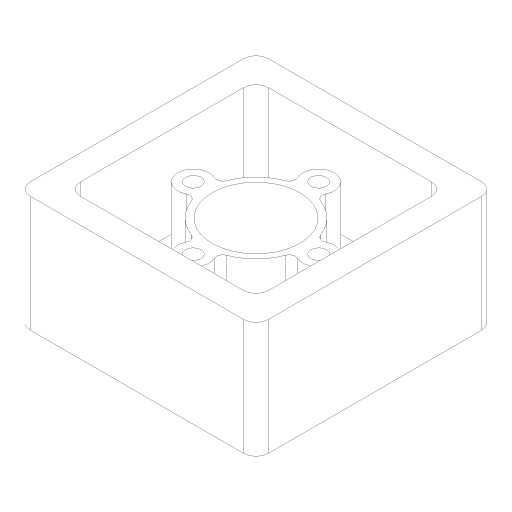
# Autodesk Inventor part: Ecoflex_mould
Saved by Autodesk Inventor 2023 (Build 270158000, 158)
## iProperties
Created: 2026-03-05
Part Number: Ecoflex_mould
Material: Generic
Document SubType Name: Modeling
Designer: ferrerx
Density: 1 g/cm^3
Appearance: Default
Author: ferrerx
Autodesk Inventor part; units mm, degrees
ref_plane "YZ Plane" through (0, 0, 0) normal (1, 0, 0) x (0, 1, 0)
ref_plane "XZ Plane" through (0, 0, 0) normal (0, 1, 0) x (-1, 0, 0)
ref_plane "XY Plane" through (0, 0, 0) normal (0, 0, 1) x (1, 0, 0)
sketch "Sketch1" plane through (0, 0, 0) normal (0, 1, 0) x (-1, 0, 0)
  circle A0 centre (0, 0) radius 7
  circle A1 centre (0, 0) radius 8
  dimension "d0" = 14
  dimension "d1" = 1
  constraints: 2 centre point, 2 coincident
  measures "d0" diameter of A0
  measures "d1" radial gap between concentric circles of A0 A1
extrude "Extrusion1" add sketch "Sketch1" along normal blind 10.5
sketch "Sketch2" plane through (0, 0, 0) normal (0, -1, 0) x (1, 0, 0)
  circle A0 centre (0, 0) radius 8
  constraints: 1 centre point, 1 coincident
extrude "Extrusion2" [suppressed]
sketch "Sketch4" plane through (0, 10.5, 0) normal (0, 1, 0) x (1, 0, 0)
  circle A0 centre (-10, 0) radius 1.25
  circle A1 centre (-10, 0) radius 2.5
  point P0 (0, 0)
  dimension "d6" = 5
  dimension "d7" = 2.5
  dimension "d8" = 10
  constraints: 2 centre point, 1 coincident
  measures "d6" diameter of A1
  measures "d7" diameter of A0
  measures "d8" distance of point (0, 0) A1.centre
extrude "Extrusion3" add sketch "Sketch4" against normal up to surface (10.5 mm away)
pattern_circular "Circular Pattern1" count 4 over 360 about axis through (0, 0, 0) along (0, 1, 0) of "Extrusion3"
fillet "Fillet1" radius 1 8 edges at (7.8875, 5.25, -1.3369) (7.8875, 5.25, 1.3369) (1.3369, 5.25, 7.8875) (-1.3369, 5.25, 7.8875) (-7.8875, 5.25, 1.3369) (-7.8875, 5.25, -1.3369) (-1.3369, 5.25, -7.8875) (1.3369, 5.25, -7.8875)
sketch "Sketch5" plane through (0, 0, 0) normal (0, -1, 0) x (1, 0, 0)
  line L0 (-15, -15) -> (15, -15)
  line L1 (15, -15) -> (15, 15)
  line L2 (15, 15) -> (-15, 15)
  line L3 (-15, 15) -> (-15, -15)
  line L4 (-15, -15) -> (15, 15) construction
  line L5 (15, -15) -> (-15, 15) construction
  point P0 (0, 0)
  dimension "d23" = 30
  dimension "d24" = 30
  constraints: 12 end point, 2 midpoint, 2 parallel, 1 horizontal, 1 perpendicular
  measures "d23" distance of L0.end L1.end
  measures "d24" distance of L0.start L0.end
extrude "Extrusion4" add sketch "Sketch5" along normal blind 4
sketch "Sketch6" plane through (0, -4, 0) normal (0, 1, 0) x (1, 0, 0)
  line L0 (15, 15) -> (15, -15) projected
  line L1 (-15, -15) -> (15, -15)
  line L2 (15, -15) -> (15, 15)
  line L3 (15, 15) -> (-15, 15)
  line L4 (-15, 15) -> (-15, -15)
  line L5 (-15, -15) -> (15, 15) construction
  line L6 (15, -15) -> (-15, 15) construction
  line L7 (-19, -19) -> (19, -19)
  line L8 (19, -19) -> (19, 19)
  line L9 (19, 19) -> (-19, 19)
  line L10 (-19, 19) -> (-19, -19)
  line L11 (-19, -19) -> (19, 19) construction
  line L12 (19, -19) -> (-19, 19) construction
  point P0 (0, 0)
  dimension "d27" = 4
  dimension "d28" = 4
  constraints: 24 end point, 4 midpoint, 4 parallel, 2 horizontal, 2 perpendicular
  measures "d27" distance between parallel lines of L4 L10
  measures "d28" distance between parallel lines of L9 L3
extrude "Extrusion5" add sketch "Sketch6" along normal blind 18.5
fillet "Fillet2" radius 2 8 edges at (-15, 7.25, -15) (15, 7.25, -15) (-15, 7.25, 15) (15, 7.25, 15) (19, 5.25, 19) (19, 5.25, -19) (-19, 5.25, 19) (-19, 5.25, -19)
body "Solid1"
